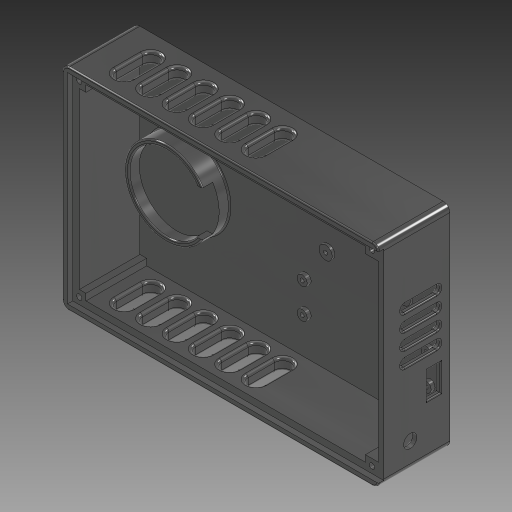
# Autodesk Inventor part: box
Saved by Autodesk Inventor 2023 (Build 270158000, 158)
## iProperties
Created: 2024-01-29
Part Number: box
Material: Všeobecné
Document SubType Name: Modeling
Designer: matej
Mass: 54.735 g
Surface Area: 398.954 cm^2
Volume: 54.735 cm^3
Density: 1 g/cm^3
Appearance: Tmavě šedá
Author: matej
## iProperties of the stored document box_3D tisk.ipt
Created: 2024-02-06
Part Number: box_3D tisk
Material: Všeobecné
Document SubType Name: Modeling
Designer: mates.exe
Mass: 54.7513 g
Surface Area: 399.126 cm^2
Volume: 54.7513 cm^3
Density: 1 g/cm^3
Appearance: Výchozí
Author: mates.exe
Autodesk Inventor part; units mm, degrees
ref_plane "YZ Plane" through (0, 0, 0) normal (1, 0, 0) x (0, 1, 0)
ref_plane "XZ Plane" through (0, 0, 0) normal (0, 1, 0) x (-1, 0, 0)
ref_plane "XY Plane" through (0, 0, 0) normal (0, 0, 1) x (1, 0, 0)
sketch "Náčrt1" plane through (0, 0, 0) normal (0, 0, 1) x (1, 0, 0)
  line L0 (-60, -40) -> (60, -40)
  line L1 (60, -40) -> (60, 40)
  line L2 (60, 40) -> (-60, 40)
  line L3 (-60, 40) -> (-60, -40)
  line L4 (-60, -40) -> (60, 40) construction
  line L5 (60, -40) -> (-60, 40) construction
  point P0 (0, 0)
  dimension "d0" = 120
  dimension "d1" = 80
  constraints: 12 end point, 2 midpoint, 2 parallel, 1 horizontal, 1 perpendicular
  measures "d0" distance of L2.end L1.end
  measures "d1" distance of L1.end L0.end
extrude "Vysunutí1" add sketch "Náčrt1" along normal blind 2
sketch "Náčrt2" plane through (0, 0, 2) normal (0, 0, 1) x (1, 0, 0)
  line L0 (60, -40) -> (60, 40) projected
  line L1 (-60, -40) -> (60, -40)
  line L2 (60, -40) -> (60, 40)
  line L3 (60, 40) -> (-60, 40)
  line L4 (-60, 40) -> (-60, -40)
  line L5 (-60, -40) -> (60, 40) construction
  line L6 (60, -40) -> (-60, 40) construction
  line L7 (-58, -38) -> (58, -38)
  line L8 (58, -38) -> (58, 38)
  line L9 (58, 38) -> (-58, 38)
  line L10 (-58, 38) -> (-58, -38)
  line L11 (-58, -38) -> (58, 38) construction
  line L12 (58, -38) -> (-58, 38) construction
  line L13 (58, 38) -> (53, 38)
  line L14 (53, 38) -> (53, 33)
  line L15 (53, 33) -> (58, 33)
  line L16 (58, 33) -> (58, 38)
  line L17 (53, 38) -> (58, 33) construction
  line L18 (58, 38) -> (53, 33) construction
  circle A0 centre (55.5, 35.5) radius 1
  circle A1 centre (55.5, -35.5) radius 1
  line L19 (53, -33) -> (53, -38)
  line L20 (58, -38) -> (58, -33)
  line L21 (58, -33) -> (53, -33)
  line L22 (53, -38) -> (58, -38)
  line L23 (53, -33) -> (58, -38) construction
  line L24 (58, -33) -> (53, -38) construction
  circle A2 centre (-55.5, 35.5) radius 1
  line L25 (-58, 38) -> (-58, 33)
  line L26 (-53, 33) -> (-53, 38)
  line L27 (-53, 38) -> (-58, 38)
  line L28 (-58, 33) -> (-53, 33)
  line L29 (-58, 38) -> (-53, 33) construction
  line L30 (-53, 38) -> (-58, 33) construction
  circle A3 centre (-55.5, -35.5) radius 1
  line L31 (-58, -33) -> (-58, -38)
  line L32 (-53, -38) -> (-53, -33)
  line L33 (-53, -33) -> (-58, -33)
  line L34 (-58, -38) -> (-53, -38)
  line L35 (-58, -33) -> (-53, -38) construction
  line L36 (-53, -33) -> (-58, -38) construction
  line L37 (53, 38) -> (-53, 38)
  line L38 (-53, 38) -> (-53, 35.5)
  line L39 (-53, 35.5) -> (53, 35.5)
  line L40 (53, 35.5) -> (53, 38)
  line L41 (-58, 33) -> (-55.5, 33)
  line L42 (-55.5, 33) -> (-55.5, -33)
  line L43 (-55.5, -33) -> (-58, -33)
  line L44 (-58, -33) -> (-58, 33)
  line L45 (-53, -38) -> (53, -38)
  line L46 (53, -38) -> (53, -35.5)
  line L47 (53, -35.5) -> (-53, -35.5)
  line L48 (-53, -35.5) -> (-53, -38)
  point P0 (0, 0)
  point P1 (60, -40)
  point P2 (-53, -35.5)
  dimension "d4" = 116
  dimension "d62" = 76
  dimension "d68" = 5
  dimension "d69" = 5
  dimension "d70" = 2
  dimension "d71" = 2.5
  dimension "d72" = 2.5
  dimension "d75" = 71
  dimension "d78" = 111
  dimension "d85" = 2.5
  dimension "d86" = 2.5
  dimension "d87" = 2.5
  constraints: 96 end point, 12 parallel, 8 midpoint, 7 horizontal, 6 perpendicular, 4 centre point, 1 vertical, 39 other
  measures "d4" distance of L9.end L8.end
  measures "d62" distance of L7.end L8.end
  measures "d68" distance of L15.end L14.end
  measures "d69" distance of L14.end L13.end
  measures "d70" diameter of A0
  measures "d71" distance from line of L8 A0.centre
  measures "d72" distance from line of L15 A0.centre
  measures "d75" distance of A0.centre A1.centre
  measures "d78" distance of A0.centre A2.centre
  measures "d85" distance of L38.end L37.end
  measures "d86" distance of L42.end L43.end
  measures "d87" distance of L46.end L45.end
extrude "Vysunutí2" add sketch "Náčrt2" along normal blind 25 contours L1 L4 L3 L0 | L10 L33 L32 L7 | L32 L47 L19 L7 | L10 L28 L42 L33 | L19 L21 L8 L7 | L10 L9 L26 L28 | L9 L14 L39 L26 | L15 L14 L9 L8
sketch "Náčrt3" plane through (60, -40, 0) normal (1, 0, 0) x (0, 0, -1)
  line L0 (-8.5, 20) -> (-3.5, 20)
  line L1 (-3.5, 20) -> (-3.5, 30)
  line L2 (-3.5, 30) -> (-8.5, 30)
  line L3 (-8.5, 30) -> (-8.5, 20)
  line L4 (-8.5, 20) -> (-3.5, 30) construction
  line L5 (-3.5, 20) -> (-8.5, 30) construction
  line L6 (0, 0) -> (0, 80) projected
  line L7 (0, 0) -> (-27, 0) projected
  line L8 (-3.5, 20) -> (-18.5, 20)
  line L9 (-18.5, 20) -> (-18.5, 60)
  line L10 (-18.5, 60) -> (-3.5, 60)
  line L11 (-3.5, 60) -> (-3.5, 20)
  line L12 (-3.5, 36.5) -> (-18.5, 36.5) construction
  line L13 (-5, 38) -> (-17, 38)
  line L14 (-17, 35) -> (-5, 35)
  arc A0 (-5, 35) -> (-5, 38) centre (-5, 36.5) ccw
  arc A1 (-17, 38) -> (-17, 35) centre (-17, 36.5) ccw
  line L15 (-17, 41) -> (-5, 41)
  line L16 (-3.5, 42.5) -> (-18.5, 42.5) construction
  line L17 (-5, 44) -> (-17, 44)
  arc A2 (-17, 44) -> (-17, 41) centre (-17, 42.5) ccw
  arc A3 (-5, 41) -> (-5, 44) centre (-5, 42.5) ccw
  line L18 (-17, 47) -> (-5, 47)
  line L19 (-3.5, 48.5) -> (-18.5, 48.5) construction
  line L20 (-5, 50) -> (-17, 50)
  arc A4 (-17, 50) -> (-17, 47) centre (-17, 48.5) ccw
  arc A5 (-5, 47) -> (-5, 50) centre (-5, 48.5) ccw
  line L21 (-17, 53) -> (-5, 53)
  line L22 (-3.5, 54.5) -> (-18.5, 54.5) construction
  line L23 (-5, 56) -> (-17, 56)
  arc A6 (-17, 56) -> (-17, 53) centre (-17, 54.5) ccw
  arc A7 (-5, 53) -> (-5, 56) centre (-5, 54.5) ccw
  point P0 (0, 40)
  point P1 (-6, 25)
  point P2 (0, 40)
  point P3 (-11, 36.5)
  point P4 (-11, 42.5)
  point P5 (-11, 48.5)
  point P6 (-11, 54.5)
  dimension "d8" = 3.5
  dimension "d9" = 5
  dimension "d10" = 10
  dimension "d63" = 20
  dimension "d127" = 15
  dimension "d128" = 40
  dimension "d129" = 3
  dimension "d130" = 5
  dimension "d133" = 6
  constraints: 52 end point, 24 point on circle, 10 point on line, 8 centre point, 5 parallel, 4 midpoint, 4 tangent, 3 perpendicular, 2 horizontal, 1 vertical, 42 other
  measures "d8" distance between parallel lines of L1 L6
  measures "d9" distance of L0.start L0.end
  measures "d10" distance of L2.end L0.start
  measures "d63" distance between parallel lines of L7 L0
  measures "d127" distance of L9.end L10.end
  measures "d128" distance of L8.end L9.end
  measures "d129" diameter of A1
  measures "d130" distance between parallel lines of L2 L14
  measures "d133" distance of L14.start L15.start
extrude "micro usb hole" cut sketch "Náčrt3" against normal blind 5 contours L3 L2 L1 L0 | A1 L13 A0 L14 | A2 L17 A3 L15 | A4 L20 A5 L18 | A6 L23 A7 L21
sketch "Náčrt4" plane through (0, 0, 2) normal (0, 0, 1) x (1, 0, 0)
  circle A0 centre (54.5, -9.3) radius 1.9
  circle A1 centre (54.5, -20.7) radius 1.9
  circle A2 centre (7.5, -9.3) radius 1.9
  circle A3 centre (7.5, -20.7) radius 1.9
  line L0 (5.5, -4.5) -> (56.5, -4.5)
  line L1 (56.5, -4.5) -> (56.5, -25.5)
  line L2 (56.5, -25.5) -> (5.5, -25.5)
  line L3 (5.5, -25.5) -> (5.5, -4.5)
  line L4 (60, -40) -> (60, 40) projected
  line L5 (58, 33) -> (58, -33) projected
  circle A4 centre (54.5, -9.3) radius 0.75
  circle A5 centre (7.5, -9.3) radius 0.75
  circle A6 centre (7.5, -20.7) radius 0.75
  circle A7 centre (54.5, -20.7) radius 0.75
  line L6 (58, -20) -> (58, -10) projected
  point P0 (0, 0)
  point P1 (56.5, -15)
  point P2 (60, 0)
  point P3 (58, 38)
  point P4 (58, -38)
  point P5 (58, 30)
  point P6 (58, -30)
  point P7 (58, -15)
  dimension "d13" = 3.8
  dimension "d14" = 3.8
  dimension "d15" = 11.4
  dimension "d16" = 3.8
  dimension "d18" = 3.8
  dimension "d19" = 51
  dimension "d20" = 2
  dimension "d21" = 2
  dimension "d22" = 21
  dimension "d23" = 4.8
  dimension "d24" = 1.5
  dimension "d25" = 1.5
  dimension "d26" = 1.5
  dimension "d27" = 1.5
  dimension "d28" = 1.5
  constraints: 8 centre point, 8 end point, 4 coincident, 3 horizontal alignment, 3 midpoint, 2 parallel, 2 vertical alignment, 1 horizontal, 1 perpendicular
  measures "d13" diameter of A0
  measures "d14" diameter of A1
  measures "d15" distance of A1.centre A0.centre
  measures "d16" diameter of A2
  measures "d18" diameter of A3
  measures "d19" distance of L0.start L0.end
  measures "d20" distance from line of L1 A0.centre
  measures "d21" distance from line of L3 A2.centre
  measures "d22" distance of L2.end L0.start
  measures "d23" distance from line of L0 A0.centre
  measures "d24" distance between parallel lines of L5 L1
  measures "d25" diameter of A4
  measures "d26" diameter of A5
  measures "d27" diameter of A6
  measures "d28" diameter of A7
extrude "rpi holder" add sketch "Náčrt4" along normal blind 1.5 contours A0 | A1 | A2 | A3
sketch "Náčrt6" plane through (60, -40, 0) normal (1, 0, 0) x (0, 0, -1)
  circle A0 centre (-15, 10) radius 2.5
  line L0 (0, 80) -> (-27, 80) projected
  line L1 (0, 0) -> (0, 80) projected
  line L2 (0, 0) -> (-27, 0) projected
  point P0 (0, 40)
  dimension "d36" = 5
  dimension "d59" = 10
  dimension "d140" = 15
  constraints: 1 centre point
  measures "d36" diameter of A0
  measures "d59" distance from line of L2 A0.centre
  measures "d140" distance from line of L1 A0.centre
extrude "rgb led hole" cut sketch "Náčrt6" against normal blind 10
sketch "Náčrt7" plane through (0, 0, 2) normal (0, 0, 1) x (1, 0, 0)
  line L0 (13.4, 33) -> (48, 33)
  line L1 (48, 33) -> (48, 1.2)
  line L2 (48, 1.2) -> (13.4, 1.2)
  line L3 (13.4, 1.2) -> (13.4, 33)
  circle A0 centre (45.5, 30.4) radius 0.75
  circle A1 centre (15.9, 30.4) radius 2.5
  circle A2 centre (15.9, 3.8) radius 0.75
  circle A3 centre (45.5, 3.8) radius 0.75
  circle A4 centre (15.9, 30.4) radius 0.75
  circle A5 centre (45.5, 30.4) radius 2.5
  circle A6 centre (45.5, 3.8) radius 2.5
  circle A7 centre (15.9, 3.8) radius 2.5
  line L4 (-58, -33) -> (-58, 33) projected
  line L5 (53, -38) -> (-53, -38) projected
  line L6 (-53, 38) -> (53, 38) projected
  circle A8 centre (7.5, -9.3) radius 1.9 projected
  line L7 (58, 33) -> (58, -33) projected
  line L8 (-53, 35.5) -> (53, 35.5) projected
  point P0 (0, 0)
  point P1 (-58, -38)
  point P2 (-58, 38)
  point P3 (58, -38)
  point P4 (13.4, 30.4)
  point P5 (13.4, 3.8)
  point P6 (48, 3.8)
  point P7 (48, 30.4)
  point P8 (-58, -30)
  point P9 (-58, 30)
  point P10 (58, 38)
  dimension "d41" = 34.6
  dimension "d42" = 31.8
  dimension "d43" = 1.5
  dimension "d44" = 5
  dimension "d45" = 29.6
  dimension "d46" = 2.5
  dimension "d47" = 2.6
  dimension "d48" = 1.5
  dimension "d49" = 1.5
  dimension "d50" = 26.6
  dimension "d51" = 1.5
  dimension "d52" = 5
  dimension "d53" = 5
  dimension "d54" = 5
  dimension "d64" = 10
  dimension "d88" = 2.5
  constraints: 8 centre point, 8 end point, 4 coincident, 2 horizontal alignment, 2 parallel, 2 vertical alignment, 1 horizontal, 1 perpendicular
  measures "d41" distance of L1.end L2.end
  measures "d42" distance of L0.end L1.end
  measures "d43" diameter of A0
  measures "d44" diameter of A1
  measures "d45" distance of A1.centre A0.centre
  measures "d46" distance from line of L1 A0.centre
  measures "d47" distance from line of L0 A0.centre
  measures "d48" diameter of A2
  measures "d49" diameter of A3
  measures "d50" distance of A0.centre A3.centre
  measures "d51" diameter of A4
  measures "d52" diameter of A5
  measures "d53" diameter of A6
  measures "d54" diameter of A7
  measures "d64" distance between parallel lines of L7 L1
  measures "d88" distance between parallel lines of L8 L0
extrude "ULN2003 holder" add sketch "Náčrt7" along normal blind 1 contours A1 | A7 | A6 | A5
sketch "Náčrt10" plane through (0, 0, 27) normal (0, 0, 1) x (1, 0, 0)
  line L0 (60, -40) -> (60, 40) projected
  line L1 (-58, 38) -> (60, 38)
  line L2 (60, 38) -> (60, -38)
  line L3 (60, -38) -> (-58, -38)
  line L4 (-58, -38) -> (-58, 38)
  line L5 (60, 40) -> (-60, 40) projected
  line L6 (-60, 40) -> (-60, -40) projected
  line L7 (-60, -40) -> (60, -40) projected
  point P0 (0, 0)
  point P1 (60, 38)
  dimension "d90" = 2
  dimension "d91" = 2
  dimension "d92" = 2
  constraints: 8 end point, 2 parallel, 1 horizontal, 1 perpendicular, 1 point on line
  measures "d90" distance between parallel lines of L5 L1
  measures "d91" distance between parallel lines of L6 L4
  measures "d92" distance between parallel lines of L7 L3
extrude "Vysunutí10" cut sketch "Náčrt10" against normal blind 2 contours L3 L4 L1 L0
sketch "Náčrt11" plane through (0, 0, 2) normal (0, 0, 1) x (1, 0, 0)
  circle A0 centre (-37.5, 0) radius 16
  line L0 (-55.5, 33) -> (-55.5, -33) projected
  point P0 (0, 0)
  dimension "d95" = 32
  dimension "d96" = 18
  constraints: 1 centre point
  measures "d95" diameter of A0
  measures "d96" distance from line of L0 A0.centre
extrude "Vysunutí11" add sketch "Náčrt11" along normal blind 8
sketch "Náčrt12" plane through (-37.5, 0, 10) normal (0, 0, 1) x (1, 0, 0)
  circle A0 centre (0, 0) radius 14.25
  line L0 (-16, -8.5) -> (16, -8.5)
  line L1 (16, -8.5) -> (16, 8.5)
  line L2 (16, 8.5) -> (-16, 8.5)
  line L3 (-16, 8.5) -> (-16, -8.5)
  line L4 (-16, -8.5) -> (16, 8.5) construction
  line L5 (16, -8.5) -> (-16, 8.5) construction
  point P0 (37.5, 0)
  point P1 (11.4373, 8.5)
  point P2 (11.4373, -8.5)
  dimension "d99" = 28.5
  dimension "d102" = 32
  dimension "d103" = 17
  constraints: 12 end point, 2 midpoint, 2 parallel, 1 centre point, 1 horizontal, 1 horizontal alignment, 1 perpendicular
  measures "d99" diameter of A0
  measures "d102" distance of L2.end L1.end
  measures "d103" distance of L1.end L0.end
extrude "Vysunutí12" cut sketch "Náčrt12" against normal blind 4 contours A0 L0 L2 | A0 L2 L1 L0 | L2 A0 | A0 L0
sketch "Náčrt15" plane through (-60, -40, 0) normal (0, -1, 0) x (1, 0, 0)
  line L0 (120, 0) -> (120, 27) projected
  line L1 (15, 8.5) -> (15, 18.5) construction
  line L2 (12, 8.5) -> (12, 18.5)
  line L3 (18, 18.5) -> (18, 8.5)
  arc A0 (12, 8.5) -> (18, 8.5) centre (15, 8.5) ccw
  arc A1 (18, 18.5) -> (12, 18.5) centre (15, 18.5) ccw
  line L4 (0, 0) -> (0, 27) projected
  line L5 (0, 27) -> (120, 27) projected
  line L6 (25, 8.5) -> (25, 18.5) construction
  line L7 (22, 8.5) -> (22, 18.5)
  line L8 (28, 18.5) -> (28, 8.5)
  arc A2 (22, 8.5) -> (28, 8.5) centre (25, 8.5) ccw
  arc A3 (28, 18.5) -> (22, 18.5) centre (25, 18.5) ccw
  line L9 (35, 8.5) -> (35, 18.5) construction
  line L10 (32, 8.5) -> (32, 18.5)
  line L11 (38, 18.5) -> (38, 8.5)
  arc A4 (32, 8.5) -> (38, 8.5) centre (35, 8.5) ccw
  arc A5 (38, 18.5) -> (32, 18.5) centre (35, 18.5) ccw
  line L12 (45, 8.5) -> (45, 18.5) construction
  line L13 (42, 8.5) -> (42, 18.5)
  line L14 (48, 18.5) -> (48, 8.5)
  arc A6 (42, 8.5) -> (48, 8.5) centre (45, 8.5) ccw
  arc A7 (48, 18.5) -> (42, 18.5) centre (45, 18.5) ccw
  line L15 (55, 8.5) -> (55, 18.5) construction
  line L16 (52, 8.5) -> (52, 18.5)
  line L17 (58, 18.5) -> (58, 8.5)
  arc A8 (52, 8.5) -> (58, 8.5) centre (55, 8.5) ccw
  arc A9 (58, 18.5) -> (52, 18.5) centre (55, 18.5) ccw
  line L18 (65, 8.5) -> (65, 18.5) construction
  line L19 (62, 8.5) -> (62, 18.5)
  line L20 (68, 18.5) -> (68, 8.5)
  arc A10 (62, 8.5) -> (68, 8.5) centre (65, 8.5) ccw
  arc A11 (68, 18.5) -> (62, 18.5) centre (65, 18.5) ccw
  point P0 (120, 13.5)
  point P1 (15, 13.5)
  point P2 (120, 13.5)
  point P3 (25, 13.5)
  point P4 (35, 13.5)
  point P5 (45, 13.5)
  point P6 (55, 13.5)
  point P7 (65, 13.5)
  dimension "d113" = 3
  dimension "d114" = 10
  dimension "d116" = 15
  dimension "d119" = 10
  constraints: 48 end point, 24 point on circle, 12 centre point, 4 tangent, 3 midpoint, 1 horizontal, 1 horizontal alignment, 1 parallel, 1 vertical, 60 other
  measures "d113" radius of A1
  measures "d114" distance of L3.start L3.end
  measures "d116" distance from line of L4 point (15, 13.5)
  measures "d119" distance of L2.start L7.start
extrude "Vysunutí14" cut sketch "Náčrt15" against normal blind 5
fillet "Zaoblení1" radius 2.5 4 edges at (60, -40, 13.5) (-60, 40, 13.5) (-60, -40, 13.5) (60, 40, 13.5)
fillet "Zaoblení2" radius 1 48 edges at (-48, -40, 13.5) (-45, -40, 21.5) (-42, -40, 13.5) (-45, -40, 5.5) (-35, -40, 21.5) (-32, -40, 13.5) (-35, -40, 5.5) (-38, -40, 13.5) (-25, -40, 21.5) (-22, -40, 13.5) (-25, -40, 5.5) (-28, -40, 13.5) (-15, -40, 21.5) (-12, -40, 13.5) (-15, -40, 5.5) (-18, -40, 13.5) (-5, -40, 21.5) (-2, -40, 13.5) (-5, -40, 5.5) (-8, -40, 13.5) (5, -40, 21.5) (8, -40, 13.5) (5, -40, 5.5) (2, -40, 13.5) (-42, -35.5, 13.5) (-45, -35.5, 21.5) (-48, -35.5, 13.5) (-45, -35.5, 5.5) (-32, -35.5, 13.5) (-35, -35.5, 21.5) (-38, -35.5, 13.5) (-35, -35.5, 5.5) (-22, -35.5, 13.5) (-25, -35.5, 21.5) (-28, -35.5, 13.5) (-25, -35.5, 5.5) (-12, -35.5, 13.5) (-15, -35.5, 21.5) (-18, -35.5, 13.5) (-15, -35.5, 5.5) (-2, -35.5, 13.5) (-5, -35.5, 21.5) (-8, -35.5, 13.5) (-5, -35.5, 5.5) (8, -35.5, 13.5) (5, -35.5, 21.5) (2, -35.5, 13.5) (5, -35.5, 5.5)
mirror "Zrcadlit2" about plane through (0, 0, 0) normal (0, 1, 0) of "Vysunutí14", "Zaoblení2"
fillet "Zaoblení3" radius 0.5 51 edges at (60, -3.5, 3.5) (60, -5, 11) (60, -3.5, 18.5) (60, -2, 11) (58, 2.5, 3.5) (58, 4, 11) (58, 2.5, 18.5) (58, 1, 11) (60, 8.5, 18.5) (60, 10, 11) (60, 8.5, 3.5) (60, 7, 11) (58, 14.5, 3.5) (58, 16, 11) (58, 14.5, 18.5) (58, 13, 11) (60, 1, 11) (60, 2.5, 18.5) (60, 4, 11) (60, 2.5, 3.5) (58, -5, 11) (58, -3.5, 3.5) (58, -2, 11) (58, -3.5, 18.5) (58, 7, 11) (58, 8.5, 3.5) (58, 10, 11) (58, 8.5, 18.5) (60, 14.5, 3.5) (60, 13, 11) (60, 14.5, 18.5) (60, 16, 11) (58, -30, 17.5) (60, -15, 3.5) (60, -10, 6) (60, -15, 8.5) (60, -20, 6) (58, -15, 3.5) (58, -10, 6) (58, -15, 8.5) (58, -20, 6) (-51.75, 0, 10) (-53.5, 0, 2) (-53.5, 0, 10) (59.0811, -39.4365, 27) (-59.2678, -39.2678, 27) (-60, 0, 27) (-59.2678, 39.2678, 27) (0, 40, 27) (59.0811, 39.4365, 27) (0, -40, 27)
equation "\"d14\" = d13"
equation "\"d16\" = d13"
equation "\"d18\" = d13"
equation "\"d26\" = d25"
equation "\"d27\" = d25"
equation "\"d28\" = d25"
equation "\"d43\" = d49"
equation "\"d44\" = d53"
equation "\"d48\" = d49"
equation "\"d51\" = d49"
equation "\"d52\" = d53"
equation "\"d54\" = d53"
